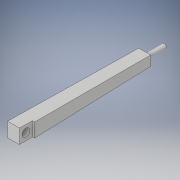
# Autodesk Inventor part: bout tournant
Saved by Autodesk Inventor 2017 (Build 210142000, 142)
## iProperties
Created: 2018-11-17
Part Number: bout tournant
Material: Generic
Document SubType Name: Modeling
Designer: Antoine Blaud
Density: 1 g/cm^3
Appearance: Default
Author: Antoine Blaud
Autodesk Inventor part; units mm, degrees
ref_plane "YZ Plane" through (0, 0, 0) normal (1, 0, 0) x (0, 1, 0)
ref_plane "XZ Plane" through (0, 0, 0) normal (0, 1, 0) x (-1, 0, 0)
ref_plane "XY Plane" through (0, 0, 0) normal (0, 0, 1) x (1, 0, 0)
sketch "Sketch1" plane through (0, 0, 0) normal (1, 0, 0) x (0, 1, 0)
  circle A0 centre (0, 0) radius 1.0033
  line L0 (-1.249071, 1.652114) -> (1.249071, 1.652114)
  line L1 (1.249071, 1.652114) -> (1.249071, -1.652114)
  line L2 (1.249071, -1.652114) -> (-1.249071, -1.652114)
  line L3 (-1.249071, -1.652114) -> (-1.249071, 1.652114)
  line L4 (-1.249071, 1.652114) -> (1.249071, -1.652114) construction
  line L5 (1.249071, 1.652114) -> (-1.249071, -1.652114) construction
  dimension "d0" = 2.0066
  dimension "d1" = 37.0909
  dimension "d2" = 2.49814
  constraints: 12 end point, 2 midpoint, 2 parallel, 1 centre point, 1 coincident, 1 horizontal, 1 perpendicular
  measures "d0" diameter of A0
  measures "d1" angle of L4 L1
  measures "d2" distance between parallel lines of L1 L3
extrude "Extrusion1" add sketch "Sketch1" along normal blind 3
sketch "Sketch2" plane through (0, -1.249071, -1.652114) normal (0, 0, -1) x (-1, 0, 0)
  line L0 (0, 0) -> (0, 2.498142)
  line L1 (-3.026642, 0) -> (0, 0)
  line L2 (0, 0) -> (0, 2.498142)
  line L3 (0, 2.498142) -> (-3.026642, 2.498142)
  line L4 (-3.026642, 2.498142) -> (-3.026642, 0)
  line L5 (-3.026642, 0) -> (0, 2.498142) construction
  line L6 (0, 0) -> (-3.026642, 2.498142) construction
  point P0 (0, 1.249071)
  point P1 (-1.513321, 1.249071)
  dimension "d5" = 50.4643
  dimension "d6" = 3.02664
  constraints: 12 end point, 2 midpoint, 2 parallel, 1 horizontal, 1 perpendicular
  measures "d5" angle of L5 L0
  measures "d6" distance between parallel lines of L4 L0
extrude "Extrusion2" add sketch "Sketch2" along normal blind 30
draft "FaceDraft1" angle 1 pull direction (0, 0, -1) faces at (1, -1.249071, -10.550705) (3.026642, 0.416357, -21.652114) (1, 1.249071, -10.550705) fixed edges at (1.513321, -1.249071, -31.652114) (3.026642, 0, -31.652114) (1.513321, 1.249071, -31.652114)
sketch "Sketch3" plane through (0, -1.249071, -31.652114) normal (0, 0, -1) x (-1, 0, 0)
  line L0 (0, 2.491731) -> (-3, -0.000251)
  line L1 (-3, 3.079469) -> (-3, -0.581327)
  line L2 (-3.026642, 0) -> (0, 0)
  line L3 (-3, 2.491731) -> (0, 0)
  circle A0 centre (-1.5, 1.245866) radius 0.5
  point P0 (0, 1.249071)
  dimension "d10" = 1
  constraints: 4 end point, 2 point on line, 1 centre point, 1 midpoint
  measures "d10" diameter of A0
extrude "Extrusion3" add sketch "Sketch3" along normal blind 5 contours A0 L3 L0 | L0 L3 A0 | L3 A0 L0 | L0 A0 L3
body "Solid1"
